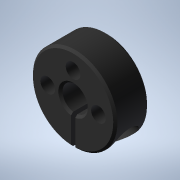
# Autodesk Inventor part: SCST6-8b
Saved by Autodesk Inventor 2021 (Build 250183000, 183)
## iProperties
Created: 2025-08-19
Part Number: SCST6-8b
Material: Generic
Catalog Web Link: www.cadenas.de
Description: SCST, PSCST, SSCST, SCSTR, PSCSTR, SSCSTR-b-Set Collars - Slit 3 Hole/3 Tap - Standard Type -
Vendor: MISUMI
Document SubType Name: Modeling
Designer: psAdmin
Manufacturer: MISUMI
Mass: 1.80633 g
Surface Area: 15.874 cm^2
Volume: 1.80633 cm^3
Density: 1 g/cm^3
Appearance: PSOLRGB-175-175-175
Category: PARTsolutions
Company: MISUMI
Title: SCST6-8
Author: Cadenas PARTsolutions
Comments: Set Collars - Slit 3 Hole/3 Tap - Standard Type -
PSOL_IDENT_0: {$CADENAS_DATA/23d-libs/misumi/metric/03_set_collars/scst/scst_b.prj},207 {VTYP=3D},{NB=SCST6-8b},{L
PSOL_IDENT_1: INA=SCST6-8},{NN=SCST, PSCST, SSCST, SCSTR, PSCSTR, SSCSTR-b},{DATE=29.11.2024 04:05:20},{GEOMDATE=1
PSOL_IDENT_2: 5.09.2021 06:06:07},{VERSION=},{LINEID=220},{WBVAR=TS,MAT,ST,BS},{WBNUMERIC=BS}  {NB=SCST6-8b},{LINA=
PSOL_IDENT_3: SCST6-8},{KT=DUMMY},{PN=SCST6-8},{TYPE=SCST},{TS=3H},{TSALG= '3H' , '3-Hole' , '3T' , '3-Tapped' },{
PSOL_IDENT_4: TSA= '3H' , '3-Hole', '3T', '3 Tap (Coarse)'},{MAT=S45C},{ST=BO},{STALG= 'BO' , 'Black Oxide' , 'ENP'
PSOL_IDENT_5: , 'Electroless Nickel Plating' },{AC=Hex Socket Head Cap Screw 1 pc.},{ACMAT=4137 Alloy Steel},{D=6
PSOL_IDENT_6: },{BS=8},{BALG= 8 , 10 },{D1=20},{M=M3},{M3D=3},{DD=3.4},{R=3.00},{W=1.0},{X=6.0},{Y=4},{P=12},{C=0.
PSOL_IDENT_7: 5},{S=3.5},{M1=-},{M13D=0},{L=12}
NB: SCST6-8b
NN: SCST, PSCST, SSCST, SCSTR, PSCSTR, SSCSTR-b
NT: Set Collars - Slit 3 Hole/3 Tap - Standard Type -
NBSYN: $PN.b
LINA: SCST6-8
CATALOG: Misumi
PN: SCST6-8
TS: 3-Hole
MAT: 1045 Carbon Steel
ST: Black Oxide
AC: Hex Socket Head Cap Screw 1 pc.
ACMAT: 4137 Alloy Steel
D: 6
BS: 8
D1: 20
M: M3
DD: 3.4
R: 3
W: 1
X: 6
Y: 4
P: 12
C: 0.5
S: 3.5
M1: -
SUPPLIER: MISUMI
ARTICLENO: SCST6-8b
BOMINFO: SCST6-8
CREATOR: CADENAS GmbH
Autodesk Inventor part; units mm, degrees
sketch "Sketch_14" plane through (0, 0, 0) normal (1, 0, 0) x (0, 1, 0)
  line L0 (0, -4) -> (0, 4)
  line L1 (0, 4) -> (9.5, 4)
  line L2 (9.5, 4) -> (10, 3.5)
  line L3 (10, 3.5) -> (10, -3.5)
  line L4 (10, -3.5) -> (9.5, -4)
  line L5 (9.5, -4) -> (0, -4)
  line L6 (0, -4) -> (0, 4)
  constraints: 14 end point
revolve "Revolution1" add sketch "Sketch_14" angle 360 about axis through (0, 0, -4) along (0, 0, -1)
sketch "Sketch_15" plane through (0, 0, 0) normal (1, 0, 0) x (0, 1, 0)
  line L0 (0, -4) -> (0, 4)
  line L1 (0, 4) -> (3.5, 4)
  line L2 (3.5, 4) -> (3, 3.5)
  line L3 (3, 3.5) -> (3, -3.5)
  line L4 (3, -3.5) -> (3.5, -4)
  line L5 (3.5, -4) -> (0, -4)
  line L6 (0, -4) -> (0, 4)
  constraints: 14 end point
revolve "Revolution2" cut sketch "Sketch_15" angle 360 about axis through (0, 0, -4) along (0, 0, -1)
sketch "Sketch_16" plane through (0, 0, 0) normal (0, 0, 1) x (1, 0, 0)
  arc A0 (-0.5, -10.9886) -> (0.5, -10.9886) centre (0, 0) ccw
  line L0 (0.5, -10.9886) -> (0.5, 0)
  line L1 (0.5, 0) -> (-0.5, 0)
  line L2 (-0.5, 0) -> (-0.5, -10.9886)
  constraints: 6 end point, 2 point on circle, 1 centre point
extrude "Extrusion1" cut sketch "Sketch_16" along normal mid plane 8
sketch "Sketch4" plane through (0, 0, -4) normal (0, 0, -1) x (-1, 0, 0)
  point P0 (-6, 0)
hole "Hole1" at (6, 0, -4) direction (0, 0, 1) diameter 3.5 depth 8
sketch "Sketch5" plane through (0, 0, -4) normal (0, 0, -1) x (-1, 0, 0)
  point P0 (6, 0)
hole "Hole2" at (-6, 0, -4) direction (0, 0, 1) diameter 3.5 depth 8
sketch "Sketch6" plane through (0, 0, -4) normal (0, 0, -1) x (-1, 0, 0)
  point P0 (0, 6)
hole "Hole3" at (0, 6, -4) direction (0, 0, 1) diameter 3.5 depth 8
sketch "Sketch_23" plane through (0, -6, 0) normal (0, 1, 0) x (1, 0, 0)
  line L0 (10, 0) -> (0, 0)
  line L1 (0, 0) -> (0, 1.7)
  line L2 (0, 1.7) -> (4, 1.7)
  line L3 (4, 1.7) -> (4, 3)
  line L4 (4, 3) -> (10, 3)
  line L5 (10, 3) -> (10, 0)
  line L6 (10, 0) -> (0, 0)
  constraints: 14 end point
revolve "Revolution3" cut sketch "Sketch_23" angle 360 about axis through (10, -6, 0) along (1, 0, 0)
sketch "Sketch8" plane through (-0.5, -9.4868, 4) normal (1, 0, 0) x (0, 0, -1)
  point P0 (4, 3.4868)
hole "Hole4" at (-0.5, -6, 0) direction (-1, 0, 0) diameter 2.459 depth 8.4303 countersink diameter 3 countersink angle 90 thread size "M3x0.5" class "6H" standard "ISO Metric profile"
ref_plane "to_bolt_XY" through (4, -6, 0) normal (1, 0, 0) x (0, 0, -1)
ref_plane "to_bolt_YZ" through (4, -6, 0) normal (0, 0, -1) x (0, 1, 0)
ref_plane "to_bolt_ZX" through (4, -6, 0) normal (0, 1, 0) x (1, 0, 0)
body "Solid1"
